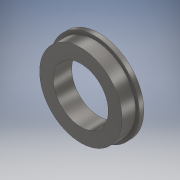
# Autodesk Inventor part: bear_f12_sa_2
Saved by Autodesk Inventor 2018 (Build 220112000, 112)
## iProperties
Created: 2018-03-04
Part Number: bear_f12_sa_2
Material: ステンレス鋼
Document SubType Name: Modeling
Designer: shun
Density: 8 g/cm^3
Appearance: 半つや出し
Author: shun
Autodesk Inventor part; units mm, degrees
ref_plane "YZ Plane" through (0, 0, 0) normal (1, 0, 0) x (0, 1, 0)
ref_plane "XZ Plane" through (0, 0, 0) normal (0, 1, 0) x (-1, 0, 0)
ref_plane "XY Plane" through (0, 0, 0) normal (0, 0, 1) x (1, 0, 0)
sketch "スケッチ1" plane through (0, 0, 0) normal (0, 0, 1) x (1, 0, 0)
  line L0 (6, 0) -> (9.75, 0)
  line L1 (9.75, 0) -> (9.75, -1)
  line L2 (6, 0) -> (6, -4)
  line L3 (6, -4) -> (9, -4)
  line L4 (9, -4) -> (9, -1)
  line L5 (9, -1) -> (9.75, -1)
  line L6 (0, -4.8) -> (0, 0.8) projected
  point P0 (0, 0)
  dimension "d0" = 6
  dimension "d1" = 3.75
  dimension "d2" = 1
  dimension "d3" = 4
  dimension "d4" = 3
  dimension "d5" = 3
  constraints: 12 end point, 2 perpendicular, 2 vertical, 1 horizontal
  measures "d0" distance of point (0, 0) L0.start
  measures "d1" distance of L0.start L0.end
  measures "d2" distance of L0.end L1.end
  measures "d3" distance of L0.start L2.end
  measures "d4" distance of L2.end L3.end
  measures "d5" distance of L3.end L4.end
revolve "回転1" add sketch "スケッチ1" angle 360 about axis through (0, -10, 0) along (0, 1, 0)
